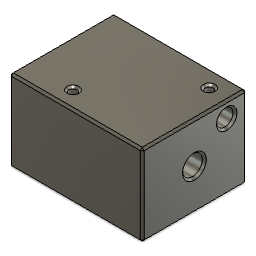
Drill Supports v2 (Autodesk Fusion 360 design; units mm, degrees)
Autodesk Fusion 360 part; units mm, degrees
sketch "Sketch1" plane through (0, 0, 0) normal (0, 1, 0) x (1, 0, 0) in component "WoaS Preamp Box Drilling Block"
  line L0 (33.5, -26.3) -> (-33.5, -26.3)
  line L1 (-33.5, -26.3) -> (-33.5, 26.3)
  line L2 (-33.5, 26.3) -> (33.5, 26.3)
  line L3 (33.5, 26.3) -> (33.5, -26.3)
  line L4 (33.5, -26.3) -> (-33.5, 26.3) construction
  line L5 (-33.5, -26.3) -> (33.5, 26.3) construction
  line L6 (0, 0) -> (-10.05, 0) construction
  line L7 (-10.05, 0) -> (-10.05, -17.7) construction
  line L8 (0, 0) -> (23.45, 0) construction
  line L9 (23.45, 0) -> (23.45, 17.5) construction
  circle A0 centre (23.45, 17.5) radius 2
  circle A1 centre (-10.05, -17.7) radius 2
  dimension "d1" = 67
  dimension "d2" = 52.6
  dimension "d3" = 10.05
  dimension "d4" = 17.7
  dimension "d5" = 23.45
  dimension "d6" = 17.5
  dimension "d7" = 4
  dimension "d8" = 4
  constraint horizontal L0
  constraint perpendicular L0 L1
  constraint parallel L0 L2
  constraint parallel L1 L3
  constraint coincident L4 L6.start
  constraint coincident L5 L6.start
  constraint coincident L6.start L8.start
  constraint horizontal L6
  constraint perpendicular L6 L7
  constraint parallel L6 L8
  constraint perpendicular L8 L9
  constraint coincident L9.end A0.centre
  constraint coincident L7.end A1.centre
  measures "d1" distance of L1.end L2.end
  measures "d2" distance of L0.end L1.end
  measures "d3" distance of L6.start L6.end
  measures "d4" distance of L6.end L7.end
  measures "d5" distance of L6.start L8.end
  measures "d6" distance of L8.end L9.end
  measures "d7" diameter of A0
  measures "d8" diameter of A1
sketch "Sketch2" plane through (0, 0, 0) normal (1, 0, 0) x (0, 0, -1) in component "WoaS Preamp Box Drilling Block"
  line L0 (-26.3, -20.5) -> (26.3, -20.5)
  line L1 (26.3, -20.5) -> (26.3, 20.5)
  line L2 (26.3, 20.5) -> (-26.3, 20.5)
  line L3 (-26.3, 20.5) -> (-26.3, -20.5)
  line L4 (-26.3, -20.5) -> (26.3, 20.5) construction
  line L5 (26.3, -20.5) -> (-26.3, 20.5) construction
  circle A0 centre (0, 0) radius 5
  line L6 (26.3, 20.5) -> (16.2834, 12.6924)
  circle A1 centre (16.2834, 12.6924) radius 4.15
  dimension "d9" = 52.6
  dimension "d10" = 41
  dimension "d11" = 10
  dimension "d12" = 12.7
  dimension "d13" = 8.3
  constraint horizontal L0
  constraint perpendicular L0 L1
  constraint parallel L0 L2
  constraint parallel L1 L3
  constraint coincident L4 A0.centre
  constraint coincident L5 A0.centre
  constraint coincident A0.centre origin
  constraint parallel L4 L6
  constraint coincident L6.end A1.centre
  measures "d9" distance of L1.end L2.end
  measures "d10" distance of L0.end L1.end
  measures "d11" diameter of A0
  measures "d12" distance of L1.end L6.end
  measures "d13" diameter of A1
extrude "Extrude1" add sketch "Sketch1" along normal mid plane 41 in component "WoaS Preamp Box Drilling Block"
extrude "Extrude2" cut sketch "Sketch2" along normal mid plane 67 contours A0 | A1 in component "WoaS Preamp Box Drilling Block"
chamfer "Chamfer1" distance 1 angle 45 6 faces at (-7.3094, 20.5, -9.2654) (-33.5, 0, 19.2) (-11.1667, 6.8333, 26.3) (-7.3094, -20.5, -9.2654) (33.5, 0, 19.2) (-11.1667, -6.8333, -26.3) in component "WoaS Preamp Box Drilling Block"
component "WoaS Preamp Box Drilling Block" placed x (1, 0, 0) y (0, 1, 0) z (0, 0, 1) at (0, 0, 0)
equation "d3 = ( 69.9 / 2 ) * 1 mm - 24.9 mm"
equation "d4 = ( 55 / 2 ) * 1 mm - 9.8 mm"
equation "d5 = ( 69.9 / 2 ) * 1 mm - 11.5 mm"
equation "d6 = ( 55 / 2 ) * 1 mm - 10 mm"
equation "d12 = ( 25.4 / 2 ) * 1 mm"
equation "d14 = ( 41 / 2 ) * 1 mm"
named bodies: "Drill Support"
